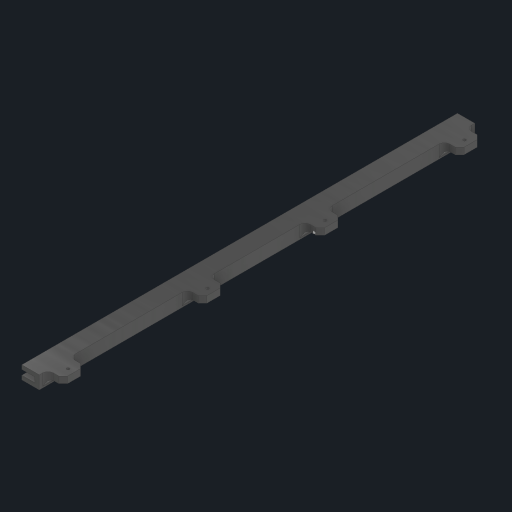
# Autodesk Inventor part: GUIA DE TAPA PRINCIPAL
Saved by Autodesk Inventor 2024.3 (Build 283343000, 343)
## iProperties
Created: 2024-06-13
Part Number: GUIA DE TAPA PRINCIPAL
Material: Generic
Document SubType Name: Modeling
Designer: Jhuliams
Density: 1 g/cm^3
Appearance: Default
Author: Jhuliams
Autodesk Inventor part; units mm, degrees
ref_plane "YZ Plane" through (0, 0, 0) normal (1, 0, 0) x (0, 1, 0)
ref_plane "XZ Plane" through (0, 0, 0) normal (0, 1, 0) x (-1, 0, 0)
ref_plane "XY Plane" through (0, 0, 0) normal (0, 0, 1) x (1, 0, 0)
sketch "Sketch1" plane through (0, 0, 0) normal (0, 0, 1) x (1, 0, 0)
  line L0 (-7.5, 2.9) -> (7.5, 2.9)
  line L1 (7.5, 2.9) -> (7.5, -2.9)
  line L2 (7.5, -2.9) -> (-7.5, -2.9)
  line L3 (-7.5, -2.9) -> (-7.5, 2.9)
  line L4 (-7.5, 2.9) -> (7.5, -2.9) construction
  line L5 (7.5, 2.9) -> (-7.5, -2.9) construction
  line L6 (-12.5, 7.5) -> (12.5, 7.5)
  line L7 (12.5, 7.5) -> (12.5, -7.5)
  line L8 (12.5, -7.5) -> (-12.5, -7.5)
  line L9 (-12.5, -7.5) -> (-12.5, 7.5)
  line L10 (-12.5, 7.5) -> (12.5, -7.5) construction
  line L11 (12.5, 7.5) -> (-12.5, -7.5) construction
  line L12 (-7.5, 7.5) -> (-7.5, -7.5)
  point P0 (0, 0)
  point P1 (-7.5, 2.9)
  dimension "d0" = 15
  dimension "d1" = 5.8
  dimension "d2" = 25
  dimension "d3" = 15
  constraints: 26 end point, 4 midpoint, 4 parallel, 3 perpendicular, 2 horizontal, 2 point on line
  measures "d0" distance of L1.end L2.end
  measures "d1" distance of L0.end L1.end
  measures "d2" distance of L7.end L8.end
  measures "d3" distance of L6.end L7.end
extrude "Extrusion1" add sketch "Sketch1" along normal blind 500 contours L12 L6 L7 L8 L2 L1 L0
ref_plane "Work Plane1" through (0, 0, 330) normal (0, 0, 1) x (1, 0, 0)
sketch "Sketch2" plane through (0, 0, 330) normal (0, 0, 1) x (1, 0, 0)
  line L0 (-5, 7.5) -> (30, 7.5)
  line L1 (30, 7.5) -> (30, -7.5)
  line L2 (30, -7.5) -> (-5, -7.5)
  line L3 (-5, -7.5) -> (-5, 7.5)
  line L4 (12.5, -7.5) -> (12.5, 7.5)
  line L5 (-5, 7.5) -> (30, -7.5) construction
  line L6 (30, 7.5) -> (-5, -7.5) construction
  line L7 (12.5, 0) -> (30, 0)
  line L8 (30, 0) -> (30, 7.5)
  line L9 (30, 7.5) -> (12.5, 7.5)
  line L10 (12.5, 7.5) -> (12.5, 0)
  line L11 (7.5, -2.9) -> (-7.5, -2.9) projected
  line L12 (-7.5, -2.9) -> (-7.5, -7.5) projected
  line L13 (-7.5, -7.5) -> (12.5, -7.5) projected
  line L14 (12.5, -7.5) -> (12.5, 7.5) projected
  line L15 (12.5, 7.5) -> (-7.5, 7.5) projected
  line L16 (-7.5, 7.5) -> (-7.5, 2.9) projected
  line L17 (-7.5, 2.9) -> (7.5, 2.9) projected
  line L18 (7.5, 2.9) -> (7.5, -2.9) projected
  point P0 (0, 0)
  point P1 (12.5, -6.5)
  point P2 (12.5, 6.5)
  point P3 (12.5, 7.5)
  point P4 (12.5, 6.5)
  point P5 (30, 0)
  dimension "d8" = 35
  constraints: 22 end point, 4 midpoint, 4 parallel, 2 horizontal, 2 perpendicular
  measures "d8" distance of L1.end L2.end
extrude "Extrusion2" add sketch "Sketch2" against normal blind 25 contours L0 L1 L7 L4
fillet "Fillet2" radius 6 3 edges at (12.5, 3.75, 305) (12.5, 0, 317.5) (12.5, 3.75, 330)
sketch "Sketch4" plane through (-7.5, 7.5, 0) normal (0, 1, 0) x (1, 0, 0)
  line L0 (20, 0) -> (0, 0) projected
  line L1 (0, 0) -> (0, -500) projected
  line L2 (20, -500) -> (0, -500) projected
  line L3 (20, -336) -> (20, -500) projected
  arc A0 (26, -330) -> (20, -336) centre (26, -336) ccw projected
  line L4 (37.5, -330) -> (26, -330) projected
  line L5 (37.5, -330) -> (37.5, -305) projected
  line L6 (26, -305) -> (37.5, -305) projected
  arc A1 (20, -299) -> (26, -305) centre (26, -299) ccw projected
  line L7 (20, 0) -> (20, -299) projected
  circle A2 centre (30.5, -317.5) radius 1.65
  line L8 (20, 0) -> (20, -500) projected
  line L9 (20, -250) -> (51.65, -250)
  circle A3 centre (30.5, -142.5) radius 1.65
  point P0 (7.5, 0)
  point P1 (20, -181)
  point P2 (20, -144)
  point P3 (37.5, -317.5)
  point P4 (37.5, -142.5)
  dimension "d16" = 3.3
  dimension "d17" = 7
  constraints: 2 centre point, 2 end point, 2 horizontal alignment, 2 midpoint, 1 equal radius, 1 horizontal, 1 vertical alignment
  measures "d16" diameter of A2
  measures "d17" distance from line of L5 A2.centre
extrude "Extrusion4" cut sketch "Sketch4" against normal through all contours A2 | A3
chamfer "Chamfer1" distance 5 angle 45 2 edges at (30, 3.75, 330) (30, 3.75, 305)
sketch "Sketch5" plane through (18.5, 0, 305) normal (0, -1, 0) x (1, 0, 0)
  line L0 (11.5, -170) -> (6.5, -175) projected
  line L1 (11.5, -170) -> (11.5, -155) projected
  line L2 (6.5, -150) -> (11.5, -155) projected
  line L3 (0, -150) -> (6.5, -150) projected
  line L4 (0, -175) -> (0, -150) projected
  line L5 (6.5, -175) -> (0, -175) projected
  circle A0 centre (4.5, -162.5) radius 1.65 projected
  circle A1 centre (4.5, 12.5) radius 1.65 projected
  line L6 (11.5, 5) -> (6.5, 0) projected
  line L7 (11.5, 20) -> (11.5, 5) projected
  line L8 (6.5, 25) -> (11.5, 20) projected
  line L9 (0, 25) -> (6.5, 25) projected
  line L10 (0, 0) -> (0, 25) projected
  line L11 (6.5, 0) -> (0, 0) projected
  circle A2 centre (4.5, 12.5) radius 2.9
  circle A3 centre (4.5, -162.5) radius 2.9
  point P0 (-18.5, -305)
  dimension "d23" = 5.8
  constraints: 2 centre point, 2 coincident, 1 equal radius
  measures "d23" diameter of A2
extrude "Extrusion5" cut sketch "Sketch5" against normal blind 3 contours A2 | A3
ref_plane "Work Plane3" through (0, 0, 250) normal (0, 0, -1) x (-1, 0, 0)
pattern_linear "Rectangular Pattern1" count 2 spacing 160 along (0, 0, 1) of "Extrusion2", "Fillet2", "Extrusion4", "Chamfer1", "Extrusion5"
mirror "Mirror1" about plane through (0, 0, 250) normal (0, 0, -1) of "Extrusion2", "Fillet2", "Extrusion4", "Chamfer1", "Extrusion5", "Rectangular Pattern1"
body "Solid1"
